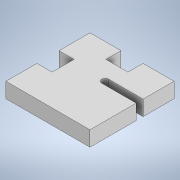
# Autodesk Inventor part: SupportV2
Saved by Autodesk Inventor 2020 (Build 240168000, 168)
## iProperties
Created: 2019-11-07
Part Number: SupportV2
Material: Générique
Document SubType Name: Modeling
Designer: erwan
Density: 1 g/cm^3
Appearance: Par défaut
Author: erwan
Autodesk Inventor part; units mm, degrees
ref_plane "YZ Plane" through (0, 0, 0) normal (1, 0, 0) x (0, 1, 0)
ref_plane "XZ Plane" through (0, 0, 0) normal (0, 1, 0) x (-1, 0, 0)
ref_plane "XY Plane" through (0, 0, 0) normal (0, 0, 1) x (1, 0, 0)
sketch "Esquisse1" plane through (0, 0, 0) normal (0, 1, 0) x (-1, 0, 0)
  line L0 (0, 0) -> (122, 0)
  line L1 (0, -122) -> (0, -77)
  line L2 (0, -77) -> (50, -77)
  arc A0 (50, -77) -> (50, -67) centre (50, -72) ccw
  line L3 (50, -67) -> (0, -67)
  line L4 (0, 0) -> (0, -67)
  line L5 (122, -122) -> (77, -122)
  line L6 (77, -122) -> (77, -100)
  line L7 (77, -100) -> (45, -100)
  line L8 (45, -100) -> (45, -122)
  line L9 (45, -122) -> (0, -122)
  line L10 (122, -122) -> (122, -77)
  line L11 (122, -77) -> (100, -77)
  line L12 (100, -77) -> (100, -45)
  line L13 (100, -45) -> (122, -45)
  line L14 (122, -45) -> (122, 0)
  dimension "d0" = 122
  dimension "d1" = 122
  dimension "d2" = 45
  dimension "d3" = 50
  dimension "d7" = 45
  dimension "d8" = 22
  dimension "d9" = 32
  dimension "d10" = 45
  dimension "d11" = 22
  dimension "d12" = 32
  constraints: 30 end point, 8 perpendicular, 3 vertical, 2 horizontal, 2 point on circle, 1 centre point, 1 point on line
  measures "d0" distance of L5.start L1.start
  measures "d1" distance of L0.end L5.start
  measures "d2" distance of L1.start L1.end
  measures "d3" distance of L1.end L2.end
  measures "d7" distance of L5.start L5.end
  measures "d8" distance of L5.end L6.end
  measures "d9" distance of L6.end L7.end
  measures "d10" distance of L5.start L10.end
  measures "d11" distance of L10.end L11.end
  measures "d12" distance of L11.end L12.end
extrude "Extrusion1" add sketch "Esquisse1" along normal blind 22
